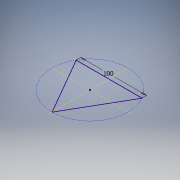
# Autodesk Inventor part: Bauteil7
Saved by Autodesk Inventor 2018.3 (Build 223284000, 284)
## iProperties
Created: 2018-09-15
Part Number: Bauteil7
Material: Generisch
Document SubType Name: Modeling
Designer: JochenAlt
Density: 1 g/cm^3
Appearance: Vorgabe
Author: JochenAlt
Autodesk Inventor part; units mm, degrees
ref_plane "YZ Plane" through (0, 0, 0) normal (1, 0, 0) x (0, 1, 0)
ref_plane "XZ Plane" through (0, 0, 0) normal (0, 1, 0) x (-1, 0, 0)
ref_plane "XY Plane" through (0, 0, 0) normal (0, 0, 1) x (1, 0, 0)
sketch "Skizze1" plane through (0, 0, 0) normal (0, 0, 1) x (1, 0, 0)
  line L0 (0, 80.5) -> (0, -80.5) construction
  line L1 (-80.5, 0) -> (80.5, 0) construction
  line L2 (0, -57.5) -> (-49.7965, 28.75)
  line L3 (-49.7965, 28.75) -> (49.7965, 28.75)
  line L4 (49.7965, 28.75) -> (0, -57.5)
  circle A0 centre (0, 0) radius 57.5 construction
  dimension "d3" = 115
  constraints: 6 end point, 1 coincident, 1 point on line, 10 other
extrude "Extrusion1" add sketch "Skizze1" against normal blind 10
